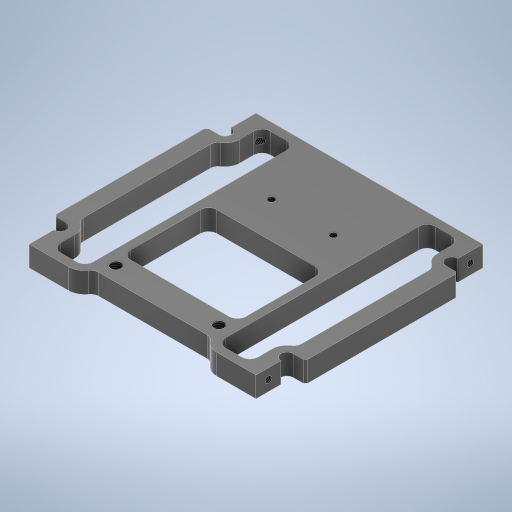
# Autodesk Inventor part: HeadLowerFrame
Saved by Autodesk Inventor 2024.2 (Build 282272000, 272)
## iProperties
Created: 2024-01-19
Part Number: HeadLowerFrame
Material: Acetal Resin, Black
Document SubType Name: Modeling
Designer: Masato Kubotera
Density: 1.425 g/cm^3
Appearance: Smooth - Black
Mass: 11.7532 g
Surface Area: 68.8447 cm^2
Volume: 8.24788 cm^3
Vendor: meviy
Author: Masato Kubotera
Autodesk Inventor part; units mm, degrees
ref_plane "YZ Plane" through (0, 0, 0) normal (1, 0, 0) x (0, 1, 0)
ref_plane "XZ Plane" through (0, 0, 0) normal (0, 1, 0) x (-1, 0, 0)
ref_plane "XY Plane" through (0, 0, 0) normal (0, 0, 1) x (1, 0, 0)
sketch "Sketch1" plane through (0, 0, 0) normal (0, 0, 1) x (1, 0, 0)
  line L0 (27.5, 27.5) -> (-27.5, 27.5) construction
  line L1 (-27.5, 27.5) -> (-27.5, -27.5)
  line L2 (-27.5, -27.5) -> (27.5, -27.5) construction
  line L3 (27.5, -27.5) -> (27.5, 27.5) construction
  line L4 (27.5, 27.5) -> (-27.5, -27.5) construction
  line L5 (-27.5, 27.5) -> (27.5, -27.5) construction
  line L6 (0, 27.5) -> (0, -27.5) construction
  line L7 (27.5, 0) -> (-27.5, 0) construction
  line L8 (18.5, 27.5) -> (18.5, 30.5)
  line L9 (18.5, 30.5) -> (-18.5, 30.5)
  line L10 (-18.5, 30.5) -> (-18.5, 27.5)
  arc A0 (-21.5, 27.5) -> (-18.5, 27.5) centre (-20, 27.5) ccw
  line L11 (18.5, -27.5) -> (18.5, -30.5)
  line L12 (18.5, -30.5) -> (-18.5, -30.5)
  line L13 (-18.5, -30.5) -> (-18.5, -27.5)
  arc A1 (-18.5, -27.5) -> (-21.5, -27.5) centre (-20, -27.5) ccw
  line L14 (-24.5, 27.5) -> (-24.5, 21.5) construction
  line L15 (0, 30.5) -> (0, 27.5) construction
  arc A2 (18.5, 27.5) -> (21.5, 27.5) centre (20, 27.5) ccw
  arc A3 (21.5, -27.5) -> (18.5, -27.5) centre (20, -27.5) ccw
  line L16 (-2.5, -10) -> (-20, -10) construction
  line L17 (-20, -10) -> (-20, 10) construction
  line L18 (-20, 10) -> (-2.5, 10) construction
  line L19 (-2.5, 10) -> (-2.5, -10) construction
  line L20 (-2.5, -10) -> (-20, 10) construction
  line L21 (-20, -10) -> (-2.5, 10) construction
  line L22 (-11.25, -7.5) -> (-11.25, 7.5) construction
  line L23 (27.5, -27.5) -> (21.5, -27.5)
  line L24 (-21.5, -27.5) -> (-27.5, -27.5)
  line L25 (-27.5, 27.5) -> (-21.5, 27.5)
  line L26 (21.5, 27.5) -> (27.5, 27.5)
  line L27 (25, -16) -> (-25, -16) construction
  line L28 (-25, -16) -> (-25, 16) construction
  line L29 (-25, 16) -> (25, 16) construction
  line L30 (25, 16) -> (25, -16) construction
  line L31 (25, -16) -> (-25, 16) construction
  line L32 (-25, -16) -> (25, 16) construction
  line L33 (21.5, -12.5) -> (21.5, 12.5) construction
  line L34 (23.5, -24) -> (-23.5, -24) construction
  line L35 (-25.5, -22) -> (-25.5, -18)
  line L36 (-23.5, -16) -> (23.5, -16)
  line L37 (25.5, -18) -> (25.5, -22)
  line L38 (25.5, -24) -> (-25.5, -16) construction
  line L39 (-25.5, -24) -> (25.5, -16) construction
  arc A4 (23.5, -24) -> (25.5, -22) centre (23.5, -22) ccw
  arc A5 (25.5, -18) -> (23.5, -16) centre (23.5, -18) ccw
  arc A6 (-25.5, -22) -> (-23.5, -24) centre (-23.5, -22) ccw
  arc A7 (-23.5, -16) -> (-25.5, -18) centre (-23.5, -18) ccw
  arc A8 (20, -24) -> (17.0665, -25.5909) centre (20, -27.5) ccw
  line L40 (15.3902, -26.5) -> (-15.3902, -26.5)
  arc A9 (-17.0665, -25.5909) -> (-20, -24) centre (-20, -27.5) ccw
  line L41 (23.5, -24) -> (20, -24)
  line L42 (-20, -24) -> (-23.5, -24)
  arc A10 (15.3902, -26.5) -> (17.0665, -25.5909) centre (15.3902, -24.5) ccw
  arc A11 (-17.0665, -25.5909) -> (-15.3902, -26.5) centre (-15.3902, -24.5) ccw
  line L43 (-25.5, 22) -> (-25.5, 18)
  line L44 (-23.5, 16) -> (23.5, 16)
  line L45 (25.5, 18) -> (25.5, 22)
  arc A12 (25.5, 22) -> (23.5, 24) centre (23.5, 22) ccw
  arc A13 (23.5, 16) -> (25.5, 18) centre (23.5, 18) ccw
  arc A14 (-23.5, 24) -> (-25.5, 22) centre (-23.5, 22) ccw
  arc A15 (-25.5, 18) -> (-23.5, 16) centre (-23.5, 18) ccw
  line L46 (15.3902, 26.5) -> (-15.3902, 26.5)
  arc A16 (-20, 24) -> (-17.0665, 25.5909) centre (-20, 27.5) ccw
  line L47 (23.5, 24) -> (20, 24)
  line L48 (-20, 24) -> (-23.5, 24)
  arc A17 (17.0665, 25.5909) -> (15.3902, 26.5) centre (15.3902, 24.5) ccw
  arc A18 (-15.3902, 26.5) -> (-17.0665, 25.5909) centre (-15.3902, 24.5) ccw
  arc A19 (17.0665, 25.5909) -> (20, 24) centre (20, 27.5) ccw
  line L49 (-0.5, -14) -> (16.5, -14)
  line L50 (18.5, -12) -> (18.5, 12)
  line L51 (16.5, 14) -> (-0.5, 14)
  line L52 (-2.5, 12) -> (-2.5, -12)
  line L53 (-2.5, -14) -> (18.5, 14) construction
  line L54 (18.5, -14) -> (-2.5, 14) construction
  arc A20 (-2.5, -12) -> (-0.5, -14) centre (-0.5, -12) ccw
  arc A21 (16.5, -14) -> (18.5, -12) centre (16.5, -12) ccw
  arc A22 (18.5, 12) -> (16.5, 14) centre (16.5, 12) ccw
  arc A23 (-0.5, 14) -> (-2.5, 12) centre (-0.5, 12) ccw
  circle A24 centre (21.5, -12.5) radius 3 construction
  arc A25 (27.5, -18) -> (25.8333, -14.7511) centre (23.5, -18) ccw
  line L55 (25, -13.1266) -> (25, 13.1266)
  arc A26 (25, -13.1266) -> (25.8333, -14.7511) centre (27, -13.1266) ccw
  arc A27 (25.8333, 14.7511) -> (27.5, 18) centre (23.5, 18) ccw
  arc A28 (25.8333, 14.7511) -> (25, 13.1266) centre (27, 13.1266) ccw
  line L56 (27.5, -27.5) -> (27.5, -18)
  line L57 (27.5, 18) -> (27.5, 27.5)
  line L58 (24.5, 27.5) -> (24.5, 21.5) construction
  point P0 (0, 0)
  point P1 (0, 0)
  point P2 (0, -0.0008)
  point P3 (-21.5, -27.5)
  point P4 (18.5, -27.5)
  point P5 (-18.5, -27.5)
  point P6 (-18.5, -27.5)
  point P7 (18.5, -27.5)
  point P8 (-11.25, 0)
  point P9 (21.5, -27.5)
  point P10 (0, -20)
  point P11 (20, -26)
  point P12 (0, 0)
  point P13 (8, 0)
  point P14 (25, -14.2919)
  dimension "d19" = 3
  dimension "d20" = 37
  dimension "d37" = 55
  dimension "d40" = 6
  dimension "d41" = 6
  dimension "d59" = 55
  dimension "d60" = 1.5
  dimension "d61" = 17.5
  dimension "d62" = 20
  dimension "d63" = 15
  dimension "d128" = 50
  dimension "d129" = 32
  dimension "d130" = 25
  dimension "d149" = 3.5
  dimension "d150" = 2
  dimension "d152" = 2
  dimension "d154" = 1
  dimension "d156" = 16.25
  dimension "d158" = 10.5
  dimension "d159" = 3.5
  dimension "d161" = 2
  dimension "d162" = 2
  dimension "d163" = 6
  constraints: 116 end point, 58 point on circle, 42 symmetric about line, 29 centre point, 26 tangent, 23 point on line, 19 midpoint, 11 collinear, 10 equal radius, 9 parallel, 8 horizontal, 8 vertical, 7 coincident, 4 perpendicular, 25 other
  measures "d19" distance of L8.start L8.end
  measures "d20" distance of L8.end L9.end
  measures "d37" distance of L2.end L3.end
  measures "d40" distance of L14.start L14.end
  measures "d41" distance between parallel lines of L10 L14
  measures "d59" distance of L3.end L1.start
  measures "d60" radius of A2
  measures "d61" distance of L17.end L18.end
  measures "d62" distance of L16.end L17.end
  measures "d63" distance of L22.start L22.end
  measures "d128" distance of L28.end L29.end
  measures "d129" distance of L27.end L28.end
  measures "d130" distance of L33.start L33.end
  measures "d149" distance between parallel lines of L30 L33
  measures "d150" distance between parallel lines of L3 L37
  measures "d152" radius of A4
  measures "d154" distance between parallel lines of L40 L2
  measures "d156" distance between parallel lines of L1 L22
  measures "d158" distance between parallel lines of L40 L36
  measures "d159" distance between parallel lines of L2 L34
  measures "d161" distance between parallel lines of L36 L49
  measures "d162" distance from line of L34 point (20, -26)
  measures "d163" diameter of A24
extrude "Extrusion1" add sketch "Sketch1" against normal blind 5
hole "M2" at (-11.25, -7.5, 0) at (-11.25, 7.5, 0) direction (0, 0, -1) diameter 1.567 end through all thread size "M2x0.4" class "6H" standard "ANSI Metric M Profile"
hole "M3" at (21.5, -12.5, 0) at (21.5, 12.5, 0) direction (0, 0, -1) diameter 2.459 end through all thread size "M3x0.5" class "6H" standard "ANSI Metric M Profile"
sketch "Sketch3" plane through (21.5, 27.5, 0) normal (0, 1, 0) x (1, 0, 0)
  line L0 (-49, 5) -> (-43, 5) projected
  line L1 (-46, 5) -> (-46, 0)
  line L2 (0, 5) -> (6, 5) projected
  line L3 (3, 5) -> (3, 0)
  line L4 (6, 0) -> (0, 0) projected
  point P0 (3, 0)
  point P1 (3, 0)
  point P2 (3, 0)
  point P3 (-46, 0)
  point P4 (-46, 2.5)
  point P5 (3, 2.5)
  constraints: 5 midpoint, 4 end point, 2 vertical, 1 coincident
hole "Side-M2" at (24.5, 27.5, -2.5) at (-24.5, 27.5, -2.5) direction (0, -1, 0) diameter 1.567 depth 6 thread size "M2x0.4" class "6H" standard "ANSI Metric M Profile"
chamfer "C0.5" distance 0.5 angle 45 4 edges at (18.5, -30.5, -2.5) (-18.5, -30.5, -2.5) (18.5, 30.5, -2.5) (-18.5, 30.5, -2.5)
mirror "Mirror1" about plane through (0, 0, 0) normal (0, 1, 0) of "Side-M2"
body "Solid1"
